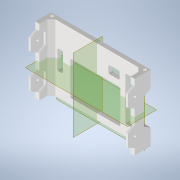
# Autodesk Inventor part: A-02
Saved by Autodesk Inventor 2022.2 (Build 262287000, 287)
## iProperties
Created: 2021-11-17
Part Number: A-02
Material: Generic
Document SubType Name: Modeling
Designer: kfcs7
Density: 1 g/cm^3
Appearance: Default
Author: kfcs7
Autodesk Inventor part; units mm, degrees
ref_plane "YZ Plane" through (0, 0, 0) normal (1, 0, 0) x (0, 1, 0)
ref_plane "XZ Plane" through (0, 0, 0) normal (0, 1, 0) x (-1, 0, 0)
ref_plane "XY Plane" through (0, 0, 0) normal (0, 0, 1) x (1, 0, 0)
ref_plane "Work Plane1" through (-121.1377, 8.8239, 118.14) normal (0, 0, -1) x (-1, 0, 0)
sketch "Sketch3" plane through (-121.1377, 8.8239, 118.14) normal (0, 0, -1) x (-1, 0, 0)
  circle A0 centre (-3.3997, 75.0001) radius 1.3753 projected
  circle A1 centre (-89.4008, 74.9992) radius 1.3739 projected
  circle A2 centre (-89.3997, 16.9995) radius 1.3745 projected
  circle A3 centre (-3.4, 17) radius 1.375 projected
  circle A4 centre (-0.0002, 78.3998) radius 0.6002 construction
  line L0 (-98.8939, 79) -> (0.0939, 79) construction
  line L1 (0.6, 78.4939) -> (0.6, 0.5061) construction
  circle A5 centre (0.0001, 0.6) radius 0.5999 construction
  line L2 (0.0939, 0) -> (-98.8939, 0) construction
  circle A6 centre (-98.7998, 0.6002) radius 0.6003 construction
  line L3 (-99.4, 0.5061) -> (-99.4, 78.4939) construction
  circle A7 centre (-98.7992, 78.3998) radius 0.6008 construction
  line L4 (0.6, 79) -> (-99.4, 79) construction
  line L5 (-99.4, 79) -> (-99.4, 0) construction
  line L6 (-99.4, 0) -> (0.6, 0) construction
  line L7 (0.6, 0) -> (0.6, 79) construction
  line L8 (-111.4, 87) -> (12.6, 87)
  line L9 (12.6, 87) -> (12.6, -8)
  line L10 (12.6, -8) -> (-111.4, -8)
  line L11 (-111.4, -8) -> (-111.4, 87)
  point P0 (-121.1377, -8.8239)
  dimension "d90" = 8
  dimension "d91" = 8
  dimension "d92" = 12
  dimension "d93" = 12
  constraints: 16 end point, 4 collinear, 4 parallel, 2 perpendicular, 1 horizontal
  measures "d90" distance between parallel lines of L0 L8
  measures "d91" distance between parallel lines of L10 L2
  measures "d92" distance between parallel lines of L11 L3
  measures "d93" distance between parallel lines of L9 L7
extrude "Extrusion1" add sketch "Sketch3" against normal blind 20 contours A0 | A1 | A2 | A3 | L8 L9 L10 L11
sketch "Sketch4" plane through (-121.1377, 8.8239, 138.14) normal (0, 0, 1) x (1, 0, 0)
  line L0 (-0.0939, 0) -> (98.8939, 0) construction
  line L1 (-12.6, -8) -> (111.4, -8) projected
  line L2 (-12.6, 87) -> (-12.6, -8) projected
  line L3 (-12.6, 4) -> (111.4, 4)
  line L4 (111.4, -8) -> (111.4, 87) projected
  point P0 (121.1377, -8.8239)
  dimension "d3" = 4
  constraints: 2 end point, 2 point on line, 1 horizontal
  measures "d3" distance between parallel lines of L3 L0
extrude "Extrusion2" cut sketch "Sketch4" against normal through all
chamfer "Chamfer1" distance 8 angle 45 2 edges at (-9.7377, 54.3239, 118.14) (-133.7377, 54.3239, 118.14)
shell "Shell1" thickness 5 removed faces 3 at (-92.4044, 40.4906, 138.14) at (-89.7377, 12.8239, 131.4734) at (-89.7377, 95.8239, 131.4734)
sketch "Sketch7" plane through (-125.7377, 12.8239, 118.14) normal (0, -1, 0) x (1, 0, 0)
  line L0 (-3, 10.0711) -> (-3, 20) projected
  line L1 (-8, 20) -> (-3, 20) projected
  line L2 (-8, 8) -> (-8, 20) projected
  line L3 (0, 0) -> (-8, 8) projected
  line L4 (108, 0) -> (0, 0) projected
  line L5 (116, 8) -> (108, 0) projected
  line L6 (116, 20) -> (116, 8) projected
  line L7 (111, 20) -> (116, 20) projected
  line L8 (111, 20) -> (111, 10.0711) projected
  line L9 (111, 10.0711) -> (105.9289, 5) projected
  line L10 (105.9289, 5) -> (2.0711, 5) projected
  line L11 (2.0711, 5) -> (-3, 10.0711) projected
  line L12 (0, 0) -> (-8, 8) projected
  line L13 (-8, 8) -> (-8, 0)
  line L14 (-8, 0) -> (0, 0)
  line L15 (2.0711, 5) -> (-3, 10.0711) projected
  point P0 (125.7377, -118.14)
  constraints: 4 end point, 1 perpendicular, 1 vertical
extrude "Extrusion5" add sketch "Sketch7" against normal blind 25 contours L3 L14 L13
sketch "Sketch8" plane through (-133.7377, 12.8239, 138.14) normal (-1, 0, 0) x (0, 0, 1)
  line L0 (-20, 0) -> (0, 0) projected
  line L1 (0, 83) -> (0, 0) projected
  line L2 (-12, 83) -> (0, 83) projected
  line L3 (-12, 25) -> (-12, 83) projected
  line L4 (-20, 25) -> (-12, 25) projected
  line L5 (-20, 0) -> (-20, 25) projected
  line L6 (-20, 25) -> (-12, 25) projected
  line L7 (-12, 25) -> (-20, 20.3812)
  line L8 (-20, 0) -> (-20, 83) projected
  line L9 (-12, 25) -> (-2.7624, 25) construction
  point P0 (-138.14, -12.8239)
  point P1 (-20, 20.3812)
  dimension "d29" = 150
  constraints: 4 end point, 1 equal length, 1 horizontal, 1 point on line
  measures "d29" angle of L7 L9
extrude "Extrusion6" cut sketch "Sketch8" along normal up to surface contours L5 L4 L7 surface through (-129.7377, 72.0739, 122.14) normal (-0.7071068, 0, -0.7071068)
sketch "Sketch12" plane through (-128.7377, 12.8239, 140.64) normal (-1, 0, 0) x (0, 0, 1)
  line L0 (-22.5, 0) -> (-2.5, 0) projected
  line L1 (-2.5, 83) -> (-2.5, 0) projected
  line L2 (-14.5, 83) -> (-2.5, 83) projected
  line L3 (-14.5, 25) -> (-14.5, 83) projected
  line L4 (-14.5, 25) -> (-22.5, 20.3812) projected
  line L5 (-2.5, 83) -> (-2.5, 0) projected
  line L6 (-2.5, 32.2376) -> (-10.5, 27.6188)
  line L7 (-10.5, 27.6188) -> (-10.5, 12.6188)
  line L8 (-10.5, 12.6188) -> (-2.5, 8)
  line L9 (-22.5, 0) -> (-22.5, 20.3812) projected
  point P0 (-140.64, -12.8239)
  point P1 (-2.5, 8)
  point P2 (-2.5, 32.2376)
  dimension "d43" = 60
  dimension "d44" = 60
  dimension "d45" = 8
  dimension "d46" = 15
  dimension "d47" = 8
  constraints: 6 end point, 2 point on line, 1 parallel
  measures "d43" angle of L1 L8
  measures "d44" angle of L1 L6
  measures "d45" distance between parallel lines of L1 L7
  measures "d46" distance of L6.end L7.end
  measures "d47" distance of L0.end L8.end
extrude "Extrusion8" cut sketch "Sketch12" along normal blind 2.5 contours L8 L7 L6 L1
sketch "Sketch15" plane through (-131.2377, 12.8239, 140.64) normal (1, 0, 0) x (0, 0, 1)
  line L0 (-10.5, -12.6188) -> (-2.5, -8) projected
  line L1 (-2.5, -8) -> (-2.5, -32.2376) projected
  line L2 (-2.5, -32.2376) -> (-10.5, -27.6188) projected
  line L3 (-10.5, -27.6188) -> (-10.5, -12.6188) projected
  line L4 (-2.5, 0) -> (-2.5, -83) projected
  line L5 (-10.5, -12.6188) -> (-2.5, -8) projected
  line L6 (-2.5, -8) -> (5.5, -12.6188)
  line L7 (5.5, -12.6188) -> (5.5, -27.6188)
  line L8 (-2.5, -32.2376) -> (-10.5, -27.6188) projected
  line L9 (5.5, -27.6188) -> (-2.5, -32.2376)
  point P0 (-140.64, 12.8239)
  dimension "d53" = 8
  dimension "d79" = 60
  dimension "d80" = 60
  dimension "d81" = 60
  dimension "d82" = 60
  dimension "d84" = 8
  constraints: 6 end point, 1 parallel
  measures "d53" distance between parallel lines of L3 L1
  measures "d79" angle of L1 L6
  measures "d80" angle of L1 L0
  measures "d81" angle of L1 L9
  measures "d82" angle of L1 L2
  measures "d84" distance between parallel lines of L7 L1
extrude "Extrusion10" add sketch "Sketch15" against normal up to surface (2.5 mm away) contours L6 L7 L9 L1
sketch "Sketch16" plane through (-131.2377, 12.8239, 140.64) normal (1, 0, 0) x (0, 0, 1)
  line L0 (-10.5, -12.6188) -> (-2.5, -8) construction
  line L1 (-2.5, -32.2376) -> (-10.5, -27.6188) construction
  line L2 (-10.5, -27.6188) -> (-10.5, -12.6188) construction
  line L3 (-2.5, 0) -> (-2.5, -83) construction
  circle A0 centre (-2.5, -20.1188) radius 1.75
  line L4 (-2.5, -32.2376) -> (5.5, -27.6188) projected
  line L5 (5.5, -27.6188) -> (5.5, -12.6188) projected
  line L6 (5.5, -12.6188) -> (-2.5, -8) projected
  point P0 (-140.64, 12.8239)
  dimension "d61" = 3.5
  constraints: 1 centre point, 1 point on line
  measures "d61" diameter of A0
extrude "Extrusion11" cut sketch "Sketch16" against normal up to next
sketch "Sketch10" plane through (-9.7377, 12.8239, 126.14) normal (0, -1, 0) x (1, 0, 0)
  line L0 (-8, -8) -> (-124, -8) projected
  line L1 (0, 0) -> (-8, -8) projected
  line L2 (0, 12) -> (0, 0) projected
  line L3 (-5, 12) -> (0, 12) projected
  line L4 (-5, 12) -> (-5, 2.0711) projected
  line L5 (-5, 2.0711) -> (-10.0711, -3) projected
  line L6 (-10.0711, -3) -> (-113.9289, -3) projected
  line L7 (-113.9289, -3) -> (-119, 2.0711) projected
  line L8 (-119, 2.0711) -> (-119, 12) projected
  line L9 (-124, 12) -> (-119, 12) projected
  line L10 (-124, -8) -> (-124, 12) projected
  line L11 (-124, 0) -> (-116, -8) construction
  circle A0 centre (-120, -4) radius 1.75
  point P0 (9.7377, -126.14)
  dimension "d37" = 3.5
  constraints: 1 centre point, 1 midpoint
  measures "d37" diameter of A0
extrude "Extrusion7" cut sketch "Sketch10" against normal blind 12 draft 2.5 contours A0
ref_plane "Work Plane3" through (-9.7377, 54.3239, 126.14) normal (0, -1, 0) x (1, 0, 0)
ref_plane "Work Plane4" through (-71.7377, 95.8239, 126.14) normal (-1, 0, 0) x (0, 0, 1)
mirror "Mirror2" about plane through (-71.7377, 95.8239, 126.14) normal (-1, 0, 0) of "Extrusion8", "Extrusion11", "Extrusion10", "Extrusion7", "Extrusion6", "Extrusion5"
mirror "Mirror3" about plane through (-9.7377, 54.3239, 126.14) normal (0, -1, 0) of "Extrusion8", "Extrusion11", "Extrusion10", "Mirror2", "Extrusion5", "Extrusion6", "Extrusion7"
chamfer "Chamfer4" distance 0.5 angle 45 4 edges at (-131.4877, 12.8239, 122.14) (-11.9877, 12.8239, 122.14) (-11.9877, 95.8239, 122.14) (-131.4877, 95.8239, 122.14)
sketch "Sketch19" plane through (-121.1377, 8.8239, 118.14) normal (0, 0, -1) x (-1, 0, 0)
  circle A0 centre (-31.4, 16.7003) radius 1.3504 construction
  circle A1 centre (-63.4002, 16.6998) radius 1.3497 construction
  circle A2 centre (-31.4, 48.7004) radius 1.3495 construction
  circle A3 centre (-63.4002, 48.7003) radius 1.3497 construction
  line L0 (-63.4002, 48.7003) -> (-31.4, 48.7003) construction
  line L1 (-31.4, 48.7003) -> (-31.4, 16.7003) construction
  line L2 (-31.4, 16.7003) -> (-63.4002, 16.7003) construction
  line L3 (-63.4002, 16.7003) -> (-63.4002, 48.7003) construction
  line L4 (-78.6501, 53.9503) -> (-16.1501, 53.9503)
  line L5 (-16.1501, 53.9503) -> (-16.1501, 11.4503)
  line L6 (-16.1501, 11.4503) -> (-78.6501, 11.4503)
  line L7 (-78.6501, 11.4503) -> (-78.6501, 53.9503)
  line L8 (-78.6501, 53.9503) -> (-16.1501, 11.4503) construction
  line L9 (-16.1501, 53.9503) -> (-78.6501, 11.4503) construction
  line L10 (-63.4002, 32.7003) -> (-47.4001, 32.7003) construction
  line L11 (-47.4001, 48.7003) -> (-47.4001, 32.7003) construction
  point P0 (-121.1377, -8.8239)
  dimension "d85" = 62.5
  dimension "d86" = 42.5
  constraints: 24 end point, 4 midpoint, 4 parallel, 4 perpendicular, 2 horizontal
  measures "d85" distance of L5.end L6.end
  measures "d86" distance of L4.end L5.end
extrude "Extrusion14" cut sketch "Sketch19" against normal through all
sketch "Sketch20" plane through (-121.1377, 8.8239, 118.14) normal (0, 0, -1) x (-1, 0, 0)
  line L0 (-86.86, 70.4) -> (-91.94, 70.4) construction
  line L1 (-86.86, 19.6) -> (-86.86, 70.4) construction
  line L2 (-91.94, 70.4) -> (-91.94, 19.6) construction
  line L3 (-91.94, 19.6) -> (-86.86, 19.6) construction
  line L4 (-84.86, 17.6) -> (-84.86, 72.4)
  line L5 (-84.86, 72.4) -> (-93.94, 72.4)
  line L6 (-93.94, 72.4) -> (-93.94, 17.6)
  line L7 (-93.94, 17.6) -> (-84.86, 17.6)
  point P0 (-121.1377, -8.8239)
  dimension "d94" = 2
  constraints: 8 end point, 3 other
  measures "d94" distance between parallel lines of L3 L7
extrude "Extrusion15" cut sketch "Sketch20" against normal through all
sketch "Sketch21" plane through (-121.1377, 8.8239, 118.14) normal (0, 0, -1) x (-1, 0, 0)
  line L0 (-2.1, 55.3) -> (-2.1, 52.125) construction
  line L1 (-2.1, 52.125) -> (-5.1, 52.125) construction
  line L2 (-5.1, 52.125) -> (-5.1, 55.3) construction
  line L3 (-5.1, 55.3) -> (-4.25, 55.3) construction
  line L4 (-4.25, 54) -> (-4.25, 55.3) construction
  line L5 (-3.95, 54) -> (-4.25, 54) construction
  line L6 (-3.95, 53.7) -> (-3.95, 54) construction
  line L7 (-2.95, 53.7) -> (-3.95, 53.7) construction
  line L8 (-2.95, 55.3) -> (-2.95, 53.7) construction
  line L9 (-2.95, 55.3) -> (-2.1, 55.3) construction
  line L10 (-5.1, 37.875) -> (-2.1, 37.875) construction
  line L11 (-2.1, 37.875) -> (-2.1, 34.7) construction
  line L12 (-2.1, 34.7) -> (-2.95, 34.7) construction
  line L13 (-2.95, 36.3) -> (-2.95, 34.7) construction
  line L14 (-3.95, 36.3) -> (-2.95, 36.3) construction
  line L15 (-3.95, 36) -> (-3.95, 36.3) construction
  line L16 (-4.25, 36) -> (-3.95, 36) construction
  line L17 (-4.25, 34.7) -> (-4.25, 36) construction
  line L18 (-4.25, 34.7) -> (-5.1, 34.7) construction
  line L19 (-5.1, 34.7) -> (-5.1, 37.875) construction
  line L20 (-2.1, 34.7) -> (-5.1, 34.7) construction
  line L21 (-5.1, 34.7) -> (-5.1, 55.3) construction
  line L22 (-5.1, 55.3) -> (-2.1, 55.3) construction
  line L23 (-2.1, 55.3) -> (-2.1, 34.7) construction
  line L24 (-0.1, 32.7) -> (-7.1, 32.7)
  line L25 (-7.1, 32.7) -> (-7.1, 57.3)
  line L26 (-7.1, 57.3) -> (-0.1, 57.3)
  line L27 (-0.1, 57.3) -> (-0.1, 32.7)
  point P0 (-121.1377, -8.8239)
  dimension "d98" = 2
  constraints: 16 end point, 4 parallel, 2 perpendicular, 1 horizontal, 3 other
  measures "d98" distance between parallel lines of L23 L27
extrude "Extrusion16" cut sketch "Sketch21" against normal through all
sketch "Sketch22" plane through (-121.1377, 8.8239, 118.14) normal (0, 0, -1) x (-1, 0, 0)
  line L0 (-68.96, 69.115) -> (-68.96, 68.815) construction
  line L1 (-68.96, 69.115) -> (-75.98, 69.115) construction
  line L2 (-75.98, 69.115) -> (-75.98, 63.315) construction
  line L3 (-74.71, 63.315) -> (-75.98, 63.315) construction
  line L4 (-74.71, 63.315) -> (-74.71, 64.315) construction
  line L5 (-74.71, 65.215) -> (-74.71, 64.315) construction
  line L6 (-69.63, 65.215) -> (-74.71, 65.215) construction
  line L7 (-69.63, 65.215) -> (-69.63, 64.315) construction
  line L8 (-69.63, 63.315) -> (-69.63, 64.315) construction
  line L9 (-65.82, 63.315) -> (-69.63, 63.315) construction
  line L10 (-65.82, 69.115) -> (-65.82, 63.315) construction
  line L11 (-65.82, 69.115) -> (-67.76, 69.115) construction
  line L12 (-67.76, 68.815) -> (-67.76, 69.115) construction
  line L13 (-68.96, 68.815) -> (-67.76, 68.815) construction
  line L14 (-67.41, 66.255) -> (-66.77, 66.255) construction
  line L15 (-67.41, 66.895) -> (-67.41, 66.255) construction
  line L16 (-66.77, 66.895) -> (-67.41, 66.895) construction
  line L17 (-66.77, 66.255) -> (-66.77, 66.895) construction
  line L18 (-69.95, 66.255) -> (-69.31, 66.255) construction
  line L19 (-69.95, 66.895) -> (-69.95, 66.255) construction
  line L20 (-69.31, 66.895) -> (-69.95, 66.895) construction
  line L21 (-69.31, 66.255) -> (-69.31, 66.895) construction
  line L22 (-72.49, 66.255) -> (-71.85, 66.255) construction
  line L23 (-72.49, 66.895) -> (-72.49, 66.255) construction
  line L24 (-71.85, 66.895) -> (-72.49, 66.895) construction
  line L25 (-71.85, 66.255) -> (-71.85, 66.895) construction
  line L26 (-75.03, 66.255) -> (-74.39, 66.255) construction
  line L27 (-75.03, 66.895) -> (-75.03, 66.255) construction
  line L28 (-74.39, 66.895) -> (-75.03, 66.895) construction
  line L29 (-74.39, 66.255) -> (-74.39, 66.895) construction
  line L30 (-65.82, 63.315) -> (-75.98, 63.315) construction
  line L31 (-75.98, 63.315) -> (-75.98, 69.115) construction
  line L32 (-75.98, 69.115) -> (-65.82, 69.115) construction
  line L33 (-65.82, 69.115) -> (-65.82, 63.315) construction
  line L34 (-77.98, 61.315) -> (-63.82, 61.315)
  line L35 (-63.82, 61.315) -> (-63.82, 71.115)
  line L36 (-63.82, 71.115) -> (-77.98, 71.115)
  line L37 (-77.98, 71.115) -> (-77.98, 61.315)
  point P0 (-121.1377, -8.8239)
  dimension "d102" = 2
  constraints: 16 end point, 4 parallel, 2 perpendicular, 1 horizontal, 3 other
  measures "d102" distance between parallel lines of L30 L34
extrude "Extrusion17" cut sketch "Sketch22" against normal through all
fillet "Fillet6" radius 2 16 edges at (-121.0378, 41.524, 120.64) (-114.0378, 41.524, 120.64) (-114.0378, 66.124, 120.64) (-121.0378, 66.124, 120.64) (-57.3178, 70.139, 120.64) (-43.1578, 70.139, 120.64) (-43.1578, 79.939, 120.64) (-57.3178, 79.939, 120.64) (-36.2778, 81.224, 120.64) (-27.1978, 81.224, 120.64) (-27.1978, 26.424, 120.64) (-36.2778, 26.424, 120.64) (-42.4877, 20.2743, 120.64) (-42.4877, 62.7743, 120.64) (-104.9877, 62.7743, 120.64) (-104.9877, 20.2743, 120.64)
equation "\"d9\" = shell_width"
equation "\"d44\" = d43"
equation "\"d79\" = d80"
equation "\"d81\" = d82"
equation "\"d84\" = d53"
equation "\"shell_width\" = 5"
body "Solid1"
